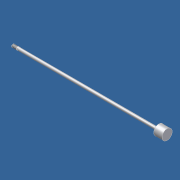
# Autodesk Inventor part: 0913-DX0_rod
Saved by Autodesk Inventor 2012 (Build 160160000, 160)
## iProperties
Category: PARTsolutions
Created: 2013-01-19
Part Number: 0913-DX0_rod
Catalog Web Link: www.cadenas.de
Description: Standard Air Cylinder_rod - Original Line - Standard Air Cylinders
Document SubType Name: Modeling
Designer: PARTsolutions
Material: Default
Density: 1 g/cm^3
Mass: 31.8618 g
Surface Area: 126.821 cm^2
Volume: 31.8618 cm^3
NB: 0913-DX0_rod
NN: Standard Air Cylinder_rod
NT: Original Line - Standard Air Cylinders
NBSYN: $PN.$COLOR1._rod
LINA: 0913-DX0_rod
PN: 0913-DX
DASH: -
BORE: 1.06250000
BOREPN: 09
STROKE: 13.000
STROKEALG: [0.001:50/0.001]
STROKE1: 13.000
ACTING: D
ACTINGALG: '' , 'Single Acting' , 'R' , 'Reverse Single Acting' , 'D' , 'Double Acting'
ACTINGPN: D
MNT: X
MNTALG: '' , 'Front Nose Mounting' , 'P' , 'Rear Pivot Mounting' , 'X' , 'Universal Pivot Mounting or Double End Mounting' , 'BF' , 'Front Block Mounting' , 'BR' , 'Rear Block Mounting for Vertical Positioning' , 'BFT' , 'Front Block Trunnion Mounting' , 'BRT' , 'Rear Block Trunnion Mounting'
MNTPN: X
DERALG: '' , 'Standard' , 'DE' , 'With Double End Rod' , 'DEH' , 'With Double End Hollow Rod'
NRALG: '' , 'N/A'
BMALG: '' , 'N/A'
COALG: '' , 'N/A'
MALG: '', 'Without Magnet', 'M', 'With Magnet'
EEL: 0
EEMAX: 37
EEALG: '', 'Without Extra Extension', 'EE', 'With Extra Extension'
EELALG: 0
EEPN1: 0.000
KALG: '', 'Standard' , 'K' , 'Ports Rotated 90deg'
QALG: '' , 'Without Side Ported Rear Head' , 'Q' , 'With Side Ported Rear Head'
YALG: '' , 'Without Pivot Bushing' , 'Y' , 'With Pivot Bushing'
FALG: '', 'Standard', 'F', 'Molycoated Body'
TALG: '' , 'Standard' , 'N' , 'Low Temperature' , 'V' , 'High Temperature'
BALG: '', 'Without Bumper' , 'B' , 'With Bumper'
HALG: '', 'N/A'
SERALG: '' , 'Without Spring Extend/Return' , 'JS' , 'With Spring Return' , 'JR' , 'With Spring Extend'
SRALG: 'C' , 'Carbon Steel Rod' , 'SR' , '303 Stainless Steel Rod' , '' , '303 Stainless Steel Rod1'
SRCON: 0
WALG: '' , 'Without Wiper' , 'W' , 'With Wiper'
EALG: '' , 'Without Special Lube and Seals' , 'E' , 'With Special Lube and Seals'
HLALG: '' , 'Wihout Low Pressure Hydraulic' , 'HL' , 'With Low Pressure Hydraulic'
STALG: '' , 'Without Switch Track' , 'T' , 'With Switch Track'
STPALG: '' , 'N/A'
PRCALG: '' , 'Without Piston Rod Clevis' , 'D-166-1' , 'With Piston Rod Clevis'
PBALG: '' , 'Without Pivot Bracket' , 'D-167' , 'With Pivot Bracket'
TLEN: 14.3135
TEXT: 0.967
SPACE: 0.552
FRAC: 184.8400
RGDACCON: R
RHCON: P
RHCONON: 1
FNUTCON: 1
RNUTCON: 1
FNUTPN: D-9
RNUTPN: D-9
FNUTTRANS: 0.0000
RNUTTRANS: 0.0000
VHOLECON: 0
A1: 1.6250
A1N: 1.0000
A1P: 1.6250
A1B: 1.8750
A4: 0.2525
A4N: 0.3750
A4P: 0.2525
A5: 0.0300
A1H: 1.500
A1NH: 0.6250
A1PH: 1.5000
A1BH: 1.1250
A1SH: 1.1250
A2H: 0.2500
A2NH: 0.2500
LENGTH: 3.8400
LENGTH1: 3.8400
LENGTH2: 4.1000
MUL: 13.0000
MUL11: 13.0000
MUL22: 33.2800
MUL33: 20.2800
MUL2: 13.0000
MUL211: 13.0000
MUL222: 2.5600
MUL233: 1.5600
SSS: 26.0000
RGLEN: 1.4025
RHLEN: 0.9990
SSS1: 14.0000
A13: 1.2190
THDLEN1: 0.5000
THD1: 0.3125
TAB: UNF
THDLEN: 0.5000
THD: 0.3125
OD: 1.0715
RODL: 16.1210
PL: 0.8710
RODDIA: 0.3120
HEX: 0.3750
RODTRANS: 0.0000
G1: 0.3440
ON: 0
G5: 0.7180
DERLEN: 15.1250
THOLE: 0.1900
WF: 0.2500
BADD: 0.0000
MADD: 0.0000
NVADD: 0.000
JRADD: 0.00000
COLOR: 0.71,0.71,0.71,0.00
GROOVE: 1
HOL: 1
D7: 0.2520
H1: 0.0000
D1: 1.1130
D1RH: 1.1110
D1P: 1.1410
D1B: 1.1130
D1N: 1.1130
D1NRH: 1.1155
D1BRH: 1.1410
D1PRH: 1.1110
BOZO: 0
HADD: 0.000
COLOR1: 0
DEFL: 0.0000
HEXL: 0.0000
SSADD: 0.0000
WFL: 0.1250
MOVE: 0.1250
KT: DUMMY
SUPPLIER: Bimba
ARTICLENO: 0913-DX0_rod
BOMINFO: 0913-DX0_rod
CREATOR: CADENAS GmbH
PSOL_IDENT_0: {\\10.0.0.242\data_v9\23d-libs\bimba\bimba\bimba_imperial\bimba_full_line\original_line_cylinders\st
PSOL_IDENT_1: andard_air_cylinders\rod.prj},278 {VTYP=3D},{NB=0913-DX0_rod},{LINA=0913-DX0_rod},{NN=Standard Air C
PSOL_IDENT_2: ylinder_rod},{DATE=11.09.2012 07:37:40},{GEOMDATE=06.09.2012 09:06:00},{VERSION=},{LINEID=10},{LINES
PSOL_IDENT_3: UBID=-1},{WBVAR=STROKE,ACTING,MNT,DER,NR,BM,CO,M,EE,EEL,K,Q,Y,F,G,T,B,H,SER,SR,NT,W,E,HL,ST,STP,PRC,
PSOL_IDENT_4: PB,COLOR1}  {NB=0913-DX0_rod},{LINA=0913-DX0_rod},{KT=DUMMY},{PN=0913-DX},{DASH=-},{BORE=1.06250000}
PSOL_IDENT_5: ,{BOREPN=09},{STROKE=13.000},{STROKEALG=[0.001:50/0.001]},{STROKE1=13.000},{ACTING=D},{ACTINGALG= ''
PSOL_IDENT_6: , 'Single Acting' , 'R' , 'Reverse Single Acting' , 'D' , 'Double Acting' },{ACTINGPN=D},{MNT=X},{M
PSOL_IDENT_7: NTALG= '' , 'Front Nose Mounting' , 'P' , 'Rear Pivot Mounting' , 'X' , 'Universal Pivot Mounting or
PSOL_IDENT_8: Double End Mounting' , 'BF' , 'Front Block Mounting' , 'BR' , 'Rear Block Mounting for Vertical Pos
PSOL_IDENT_9: itioning' , 'BFT' , 'Front Block Trunnion Mounting' , 'BRT' , 'Rear Block Trunnion Mounting' },{TYPE
PSOL_IDENT_10: =},{MNTPN=X},{DER=},{DERALG= '' , 'Standard' , 'DE' , 'With Double End Rod' , 'DEH' , 'With Double E
PSOL_IDENT_11: nd Hollow Rod' },{NR=},{NRALG= '' , 'N/A' },{NRPN=},{BM=},{BMALG= '' , 'N/A' },{BMPN=},{CO=},{COALG=
PSOL_IDENT_12: '' , 'N/A' },{M=},{MALG= '', 'Without Magnet', 'M', 'With Magnet' },{EE=},{EEL=0},{EEMAX=37},{EEALG
PSOL_IDENT_13: = '', 'Without Extra Extension', 'EE', 'With Extra Extension' },{EELALG=0},{EEPN=},{EEPN1=0.000},{K=
PSOL_IDENT_14: },{KALG= '', 'Standard' , 'K' , 'Ports Rotated 90deg' },{KPN=},{Q=},{QALG= '' , 'Without Side Ported
PSOL_IDENT_15: Rear Head' , 'Q' , 'With Side Ported Rear Head' },{QPN=},{Y=},{YALG= '' , 'Without Pivot Bushing' ,
PSOL_IDENT_16: 'Y' , 'With Pivot Bushing' },{YPN=},{F=},{FALG= '', 'Standard', 'F', 'Molycoated Body' },{FPN=},{G=
PSOL_IDENT_17: },{GPN=},{T=},{TALG= '' , 'Standard' , 'N' , 'Low Temperature' , 'V' , 'High Temperature' },{NPN=},{
PSOL_IDENT_18: VPN=},{B=},{BALG= '', 'Without Bumper' , 'B' , 'With Bumper' },{BPN=},{H=},{HALG= '', 'N/A' },{HPN=}
PSOL_IDENT_19: ,{SER=},{SERALG= '' , 'Without Spring Extend/Return' , 'JS' , 'With Spring Return' , 'JR' , 'With Sp
PSOL_IDENT_20: ring Extend' },{SR=},{SRALG= 'C' , 'Carbon Steel Rod' , 'SR' , '303 Stainless Steel Rod' , '' , '303
PSOL_IDENT_21: Stainless Steel Rod1' },{SRPN=},{SRCON=0},{NT=},{NTPN=},{W=},{WALG= '' , 'Without Wiper' , 'W' , 'W
PSOL_IDENT_22: ith Wiper' },{WPN=},{E=},{EALG= '' , 'Without Special Lube and Seals' , 'E' , 'With Special Lube and
PSOL_IDENT_23: Seals' },{EPN=},{HL=},{HLALG= '' , 'Wihout Low Pressure Hydraulic' , 'HL' , 'With Low Pressure Hydr
PSOL_IDENT_24: aulic' },{ST=},{STALG= '' , 'Without Switch Track' , 'T' , 'With Switch Track' },{STP=},{STPALG= ''
PSOL_IDENT_25: , 'N/A' },{STPN=},{PRC=},{PRCALG= '' , 'Without Piston Rod Clevis' , 'D-166-1' , 'With Piston Rod Cl
PSOL_IDENT_26: evis' },{PRCPN=},{PB=},{PBALG= '' , 'Without Pivot Bracket' , 'D-167' , 'With Pivot Bracket' },{PBPN
PSOL_IDENT_27: =},{TLEN=14.3135},{TEXT=0.966667},{SPACE=0.552381},{FRAC=184.8400},{RGCON=},{RGDACCON=R},{RHCON=P},{
PSOL_IDENT_28: RHCONON=1},{RHACCON=},{FNUTCON=1},{RNUTCON=1},{FNUTPN=D-9},{RNUTPN=D-9},{FNUTTRANS=0.0000},{RNUTTRAN
PSOL_IDENT_29: S=0.0000},{VHOLECON=0},{A1=1.6250},{A1N=1.0000},{A1P=1.6250},{A1B=1.8750},{A4=0.2525},{A4N=0.3750},{
PSOL_IDENT_30: A4P=0.2525},{A5=0.0300},{A1H=1.5},{A1NH=0.6250},{A1PH=1.5000},{A1BH=1.1250},{A1SH=1.1250},{A2H=0.250
PSOL_IDENT_31: 0},{A2NH=0.2500},{LENGTH=3.8400},{LENGTH1=3.8400},{LENGTH2=4.1000},{MUL=13.0000},{MUL11=13.0000},{MU
PSOL_IDENT_32: L22=33.2800},{MUL33=20.2800},{MUL2=13.0000},{MUL211=13.0000},{MUL222=2.5600},{MUL233=1.5600},{SSS=26
PSOL_IDENT_33: .0000},{RGLEN=1.4025},{RHLEN=0.9990},{SSS1=14.0000},{A13=1.2190},{THDLEN1=0.5000},{THD1=0.3125},{TAB
PSOL_IDENT_34: =UNF},{THDLEN=0.5000},{THD=0.3125},{OD=1.0715},{RODL=16.1210},{PL=0.8710},{RODDIA=0.3120},{HEX=0.375
PSOL_IDENT_35: 0},{RODTRANS=0.0000},{G1=0.3440},{ON=0},{G5=0.7180},{DERLEN=15.1250},{THOLE=0.1900},{WF=0.2500},{BAD
PSOL_IDENT_36: D=0.0000},{MADD=0.0000},{NVADD=0.000},{JRADD=0.00000},{COLOR=0.71,0.71,0.71,0.00},{GROOVE=1},{HOL=1}
PSOL_IDENT_37: ,{D7=0.2520},{H1=0.0000},{D1=1.1130},{D1RH=1.1110},{D1P=1.1410},{D1B=1.1130},{D1N=1.1130},{D1NRH=1.1
PSOL_IDENT_38: 155},{D1BRH=1.1410},{D1PRH=1.1110},{BOZO=0},{HADD=0.000},{COLOR1=0},{DEFL=0.0000},{HEXL=0.0000},{SSA
PSOL_IDENT_39: DD=0.0000},{WFL=0.1250},{MOVE=0.1250}
Title: 0913-DX0_rod
Author: Cadenas PARTsolutions
Comments: Original Line - Standard Air Cylinders
Autodesk Inventor part; units mm, degrees
sketch "Sketch_1" plane through (0, 0, 0) normal (0, 0, 1) x (1, 0, 0)
  line L0 (393.5984, 0) -> (-3.175, 0)
  line L1 (-3.175, 0) -> (-3.175, 3.9624)
  line L2 (-3.175, 3.9624) -> (371.475, 3.9624)
  line L3 (371.475, 3.9624) -> (371.475, 13.5572)
  line L4 (371.475, 13.5572) -> (393.5984, 13.5572)
  line L5 (393.5984, 13.5572) -> (393.5984, 0)
  line L6 (393.5984, 0) -> (-3.175, 0)
  constraints: 14 end point
revolve "Revolution1" add sketch "Sketch_1" angle 360 about axis through (393.5984, 0, 0) along (1, 0, 0)
sketch "Sketch_3" plane through (0, 0, 0) normal (0, 0, 1) x (1, 0, 0)
  line L0 (-3.175, 0) -> (-15.875, 0)
  line L1 (-15.875, 0) -> (-15.875, 3.3388)
  line L2 (-15.875, 3.3388) -> (-15.2451, 3.9688)
  line L3 (-15.2451, 3.9688) -> (-3.175, 3.9688)
  line L4 (-3.175, 3.9688) -> (-3.175, 0)
  line L5 (-3.175, 0) -> (-15.875, 0)
  constraints: 12 end point
revolve "Revolution2" add sketch "Sketch_3" angle 360 about axis through (-3.175, 0, 0) along (1, 0, 0)
thread "Thread1" size "5/16-20 UN" class "3A" standard "ANSI Unified Screw Threads" full length
sketch "Sketch_10" plane through (-3.175, 0, 0) normal (1, 0, 0) x (0, 0, -1)
  line L0 (-7.9248, 7.9248) -> (-7.9248, -7.9248)
  line L1 (-7.9248, -7.9248) -> (7.9248, -7.9248)
  line L2 (7.9248, -7.9248) -> (7.9248, 7.9248)
  line L3 (7.9248, 7.9248) -> (-7.9248, 7.9248)
  line L4 (-3.175, 3.9624) -> (-3.175, -3.9624)
  line L5 (-3.175, -3.9624) -> (3.175, -3.9624)
  line L6 (3.175, -3.9624) -> (3.175, 3.9624)
  line L7 (3.175, 3.9624) -> (-3.175, 3.9624)
  constraints: 16 end point
extrude "Extrusion1" cut sketch "Sketch_10" along normal blind 3.175
ref_plane "rod_cp_XY" through (0, 0, 0) normal (1, 0, 0) x (0, 0, -1)
ref_plane "rod_cp_YZ" through (0, 0, 0) normal (0, 0, -1) x (0, 1, 0)
ref_plane "rod_cp_ZX" through (0, 0, 0) normal (0, 1, 0) x (1, 0, 0)
ref_plane "to_rod_clevis_XY" through (-15.875, 0, 0) normal (1, 0, 0) x (0, 0, -1)
ref_plane "to_rod_clevis_YZ" through (-15.875, 0, 0) normal (0, 0, -1) x (0, 1, 0)
ref_plane "to_rod_clevis_ZX" through (-15.875, 0, 0) normal (0, 1, 0) x (1, 0, 0)
ref_plane "rl2_XY" through (-3.175, 0, 0) normal (1, 0, 0) x (0, 0, -1)
ref_plane "rl2_YZ" through (-3.175, 0, 0) normal (0, 0, -1) x (0, 1, 0)
ref_plane "rl2_ZX" through (-3.175, 0, 0) normal (0, 1, 0) x (1, 0, 0)
ref_plane "rl1_XY" through (-15.875, 0, 0) normal (1, 0, 0) x (0, 0, -1)
ref_plane "rl1_YZ" through (-15.875, 0, 0) normal (0, 0, -1) x (0, 1, 0)
ref_plane "rl1_ZX" through (-15.875, 0, 0) normal (0, 1, 0) x (1, 0, 0)
ref_plane "thd1_XY" through (-15.875, 3.9688, 0) normal (1, 0, 0) x (0, 0, -1)
ref_plane "thd1_YZ" through (-15.875, 3.9688, 0) normal (0, 0, -1) x (0, 1, 0)
ref_plane "thd1_ZX" through (-15.875, 3.9688, 0) normal (0, 1, 0) x (1, 0, 0)
ref_plane "thd2_XY" through (-15.875, -3.9688, 0) normal (1, 0, 0) x (0, 0, -1)
ref_plane "thd2_YZ" through (-15.875, -3.9688, 0) normal (0, 0, -1) x (0, 1, 0)
ref_plane "thd2_ZX" through (-15.875, -3.9688, 0) normal (0, 1, 0) x (1, 0, 0)
ref_plane "dia1_XY" through (-3.175, 3.9624, 0) normal (1, 0, 0) x (0, 0, -1)
ref_plane "dia1_YZ" through (-3.175, 3.9624, 0) normal (0, 0, -1) x (0, 1, 0)
ref_plane "dia1_ZX" through (-3.175, 3.9624, 0) normal (0, 1, 0) x (1, 0, 0)
ref_plane "dia2_XY" through (-3.175, -3.9624, 0) normal (1, 0, 0) x (0, 0, -1)
ref_plane "dia2_YZ" through (-3.175, -3.9624, 0) normal (0, 0, -1) x (0, 1, 0)
ref_plane "dia2_ZX" through (-3.175, -3.9624, 0) normal (0, 1, 0) x (1, 0, 0)
ref_plane "wf1_XY" through (-3.175, 0, 0) normal (1, 0, 0) x (0, 0, -1)
ref_plane "wf1_YZ" through (-3.175, 0, 0) normal (0, 0, -1) x (0, 1, 0)
ref_plane "wf1_ZX" through (-3.175, 0, 0) normal (0, 1, 0) x (1, 0, 0)
ref_plane "wf2_XY" through (0, 0, 0) normal (1, 0, 0) x (0, 0, -1)
ref_plane "wf2_YZ" through (0, 0, 0) normal (0, 0, -1) x (0, 1, 0)
ref_plane "wf2_ZX" through (0, 0, 0) normal (0, 1, 0) x (1, 0, 0)
ref_plane "hh1_XY" through (421.3606, 0, 0) normal (0, 0, 1) x (1, 0, 0)
ref_plane "hh1_YZ" through (421.3606, 0, 0) normal (1, 0, 0) x (0, 1, 0)
ref_plane "hh1_ZX" through (421.3606, 0, 0) normal (0, 1, 0) x (0, 0, 1)
ref_plane "hh2_XY" through (427.7614, 0, 0) normal (0, 0, 1) x (1, 0, 0)
ref_plane "hh2_YZ" through (427.7614, 0, 0) normal (1, 0, 0) x (0, 1, 0)
ref_plane "hh2_ZX" through (427.7614, 0, 0) normal (0, 1, 0) x (0, 0, 1)
ref_plane "dia12_XY" through (0, 0, 14.1351) normal (1, 0, 0) x (0, 0, -1)
ref_plane "dia12_YZ" through (0, 0, 14.1351) normal (0, 0, -1) x (0, 1, 0)
ref_plane "dia12_ZX" through (0, 0, 14.1351) normal (0, 1, 0) x (1, 0, 0)
ref_plane "dia22_XY" through (0, 0, -14.1351) normal (1, 0, 0) x (0, 0, -1)
ref_plane "dia22_YZ" through (0, 0, -14.1351) normal (0, 0, -1) x (0, 1, 0)
ref_plane "dia22_ZX" through (0, 0, -14.1351) normal (0, 1, 0) x (1, 0, 0)
ref_plane "wfw1_XY" through (-3.175, 0, -3.175) normal (0, 1, 0) x (1, 0, 0)
ref_plane "wfw1_YZ" through (-3.175, 0, -3.175) normal (1, 0, 0) x (0, 0, -1)
ref_plane "wfw1_ZX" through (-3.175, 0, -3.175) normal (0, 0, -1) x (0, 1, 0)
ref_plane "wfw2_XY" through (-3.175, 0, 3.175) normal (0, 1, 0) x (1, 0, 0)
ref_plane "wfw2_YZ" through (-3.175, 0, 3.175) normal (1, 0, 0) x (0, 0, -1)
ref_plane "wfw2_ZX" through (-3.175, 0, 3.175) normal (0, 0, -1) x (0, 1, 0)
body "Solid1"
